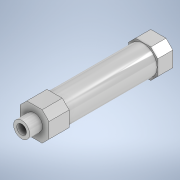
# Autodesk Inventor part: airclinder_30
Saved by Autodesk Inventor 2022 (Build 260153070, 153G)
## iProperties
Created: 2022-08-24
Part Number: airclinder_30
Material: アルミニウム 6061-AHC
Document SubType Name: Modeling
Designer: zegi
Density: 2.7 g/cm^3
Appearance: アルミニウム - ダーク
Author: zegi
Autodesk Inventor part; units mm, degrees
ref_plane "YZ Plane" through (0, 0, 0) normal (1, 0, 0) x (0, 1, 0)
ref_plane "XZ Plane" through (0, 0, 0) normal (0, 1, 0) x (-1, 0, 0)
ref_plane "XY Plane" through (0, 0, 0) normal (0, 0, 1) x (1, 0, 0)
sketch "スケッチ1" plane through (0, 0, 0) normal (0, 0, 1) x (1, 0, 0)
  line L0 (0, 0) -> (18, 0)
  line L1 (18, 0) -> (18, 18)
  line L2 (18, 18) -> (0, 18)
  line L3 (0, 18) -> (0, 0)
  line L4 (0, 13.7574) -> (4.2426, 18)
  line L5 (0, 13.7574) -> (6, 13.7574) construction
  line L6 (4.2426, 0) -> (0, 4.2426)
  line L7 (18, 4.2426) -> (13.7574, 0)
  line L8 (13.7574, 18) -> (18, 13.7574)
  point P0 (0, 9)
  point P1 (9, 18)
  point P2 (9, 9)
  dimension "d0" = 18
  dimension "d1" = 18
  dimension "d2" = 45
  dimension "d3" = 3
  dimension "d13" = 9
  dimension "d14" = 9
  dimension "d17" = 360
  constraints: 18 end point, 2 horizontal, 2 midpoint, 2 parallel, 2 point on line, 1 perpendicular, 13 other
  measures "d0" distance of L2.end L1.end
  measures "d1" distance of L1.end L0.end
  measures "d2" angle of L5 L4
  measures "d3" distance from line of L2.end L4
  measures "d13" distance from line of L2 point (9, 9)
  measures "d14" distance from line of L3 point (9, 9)
extrude "押し出し1" add sketch "スケッチ1" along normal blind 9.5 contours L6 L3 L4 L2 L8 L1 L7 L0
sketch "スケッチ2" plane through (0, 0, 9.5) normal (0, 0, 1) x (1, 0, 0)
  line L0 (0, 0) -> (13.7574, 0) projected
  line L1 (0, 13.7574) -> (0, 0) projected
  circle A0 centre (9, 9) radius 8.7
  point P0 (9, 0)
  point P1 (5.6569, 0)
  point P2 (12.3431, 0)
  point P3 (0, 9.7071)
  point P4 (0, 5.6569)
  point P5 (18, 0)
  point P6 (0, 18)
  dimension "d10" = 17.4
  constraints: 2 point on line, 1 centre point, 1 coincident
  measures "d10" diameter of A0
extrude "押し出し2" add sketch "スケッチ2" along normal blind 55
sketch "スケッチ3" plane through (9, 9, 64.5) normal (0, 0, 1) x (1, 0, 0)
  circle A0 centre (0, 0) radius 8.7 projected
  line L0 (4.7574, 9) -> (-4.7574, 9) projected
  line L1 (-4.7574, 9) -> (-9, 4.7574) projected
  line L2 (-9, 4.7574) -> (-9, -4.7574) projected
  line L3 (-9, -4.7574) -> (-4.7574, -9) projected
  line L4 (-4.7574, -9) -> (4.7574, -9) projected
  line L5 (4.7574, -9) -> (9, -4.7574) projected
  line L6 (9, -4.7574) -> (9, 4.7574) projected
  line L7 (9, 4.7574) -> (4.7574, 9) projected
  point P0 (-9, -9)
extrude "押し出し3" add sketch "スケッチ3" along normal blind 12.5 contours A0 | L7 L6 L5 L4 L3 L2 L1 L0
sketch "スケッチ4" plane through (9, 9, 77) normal (0, 0, 1) x (1, 0, 0)
  circle A0 centre (0, 0) radius 8.7 projected
  circle A1 centre (0, 0) radius 5
  point P0 (-9, -9)
  dimension "d21" = 10
  constraints: 1 centre point, 1 coincident
  measures "d21" diameter of A1
extrude "押し出し4" add sketch "スケッチ4" along normal blind 8 contours A1
sketch "スケッチ5" plane through (9, 9, 85) normal (0, 0, 1) x (1, 0, 0)
  circle A0 centre (0, 0) radius 5 projected
  circle A1 centre (0, 0) radius 3
  point P0 (-9, -9)
  dimension "d24" = 6
  constraints: 1 centre point, 1 coincident
  measures "d24" diameter of A1
extrude "押し出し5" cut sketch "スケッチ5" against normal blind 70 contours A1
equation "\"d13\" = 0.5 * d1"
